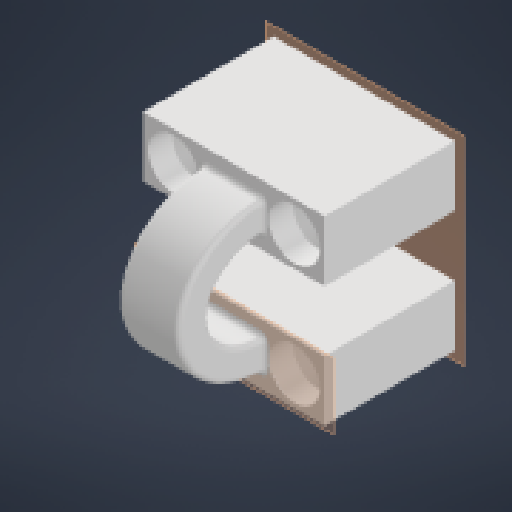
# Autodesk Inventor part: tm_top
Saved by Autodesk Inventor 2027 (Build 310192060, 192F)
## iProperties
Created: 2026-05-29
Part Number: tm_top
Material: Generic
Document SubType Name: Modeling
Designer: jacob
Density: 1 g/cm^3
Appearance: Default
Mass: 5.14574 g
Surface Area: 35.508 cm^2
Volume: 5.14574 cm^3
Author: jacob
Autodesk Inventor part; units mm, degrees
ref_plane "YZ Plane" through (0, 0, 0) normal (1, 0, 0) x (0, 1, 0)
ref_plane "XZ Plane" through (0, 0, 0) normal (0, 1, 0) x (-1, 0, 0)
ref_plane "XY Plane" through (0, 0, 0) normal (0, 0, 1) x (1, 0, 0)
ref_plane "Work Plane3" through (0, 0, 0) normal (0, 0, 1) x (1, 0, 0)
sketch "base_sketch" plane through (0, 0, 0) normal (0, 0, 1) x (1, 0, 0)
  line L0 (18.75, 18.75) -> (-18.75, 18.75) projected
  circle A0 centre (12.5, 12.5) radius 3.25
  circle A1 centre (-12.5, 12.5) radius 3.25
  line L1 (-18.75, 18.75) -> (-18.75, 6.25)
  line L2 (-18.75, 6.25) -> (18.75, 6.25)
  line L3 (18.75, 6.25) -> (18.75, 18.75)
  line L4 (0, 0) -> (-18.75, 0)
  line L5 (18.75, -18.75) -> (-18.75, -18.75)
  circle A2 centre (12.5, -12.5) radius 3.25
  circle A3 centre (-12.5, -12.5) radius 3.25
  line L6 (-18.75, -18.75) -> (-18.75, -6.25)
  line L7 (-18.75, -6.25) -> (18.75, -6.25)
  line L8 (18.75, -6.25) -> (18.75, -18.75)
  dimension "d11" = 12.5
  dimension "d41" = 6.5
  dimension "d42" = 6.5
  constraints: 16 end point, 6 symmetric about line, 4 centre point, 3 perpendicular, 1 point on line, 1 vertical, 2 other
  measures "d11" distance of L0.end L1.end
  measures "d41" diameter of A0
  measures "d42" diameter of A1
extrude "base" add sketch "base_sketch" along normal blind 27
sketch "Sketch7" plane through (0, 0, 27) normal (0, 0, 1) x (1, 0, 0)
  line L0 (-6.25, 15.5) -> (6.25, 15.5)
  line L1 (6.25, 15.5) -> (6.25, 9.25)
  line L2 (6.25, 9.25) -> (-6.25, 9.25)
  line L3 (-6.25, 9.25) -> (-6.25, 15.5)
  line L4 (-18.75, 18.75) -> (-18.75, 6.25)
  line L5 (0, 0) -> (-18.75, 0)
  line L6 (18.75, 18.75) -> (-18.75, 18.75) projected
  line L7 (-18.75, 6.25) -> (18.75, 6.25) projected
  dimension "d15" = 12.5
  dimension "d16" = 12.5
  dimension "d18" = 6.25
  dimension "d20" = 9.25
  constraints: 12 end point, 2 horizontal, 2 parallel, 1 perpendicular
  measures "d15" distance between parallel lines of L1 L3
  measures "d16" distance between parallel lines of L4 L3
  measures "d18" distance of L0.end L1.end
  measures "d20" distance between parallel lines of L7 L0
sketch "Sketch8" plane through (-18.75, 6.25, 0) normal (-1, 0, 0) x (0, 0, 1)
  line L0 (27, 3) -> (27, 9.25) projected
  ellipse E0 centre (27, -6.25) end of major axis (27, 4.125) minor radius 12.5
  line L1 (0, 0) -> (27, 0) projected
  dimension "d32" = 12.5
  dimension "d33" = 10.375
  dimension "d34" = 6.25
  dimension "d50" = 0
  constraints: 2 other
  measures "d34" distance from line of L1 point (27, -6.25)
  measures "d50" horizontal distance of L1.end point (27, -6.25)
sweep "Sweep4" add profiles "Sketch7" path "Sketch8" separate body path curves E0
ref_plane "Work Plane6" through (0, 0, 27) normal (0, 0, 1) x (1, 0, 0)
split "Split4" plane through (0, 0, 27) removes the side toward (0, 0, -1) bodies 2
combine bodies "Combine1" operation type add bodies to combine 2 1
fillet "Fillet1" radius 1 12 edges at (6.25, -12.375, 27) (0, -15.5, 27) (0, -9.25, 27) (-6.25, -12.375, 27) (6.25, 0, 44.625) (6.25, 0, 38.375) (-6.25, 0, 44.625) (-6.25, 0, 38.375) (0, 15.5, 27) (-6.25, 12.375, 27) (0, 9.25, 27) (6.25, 12.375, 27)
ref_plane "Work Plane7" through (0, 0, 0) normal (0, 0, 1) x (1, 0, 0)
sketch "Sketch12" plane through (-18.75, -6.25, 27) normal (0, 0, 1) x (1, 0, 0)
  circle A0 centre (6.25, 18.75) radius 3.25 projected
  circle A1 centre (6.25, -6.25) radius 3.25 projected
  circle A2 centre (31.25, -6.25) radius 3.25 projected
  circle A3 centre (31.25, 18.75) radius 3.25 projected
  point P0 (18.75, 6.25)
hole "Hole1" at (-12.5, -12.5, 27) at (-12.5, 12.5, 27) at (12.5, -12.5, 27) at (12.5, 12.5, 27) direction (0, 0, -1) diameter 10.5 depth 21 tip angle 118 bodies 2
equation "\"d42\" = d41"
equation "\"d16\" = d15"
body "Solid7"
